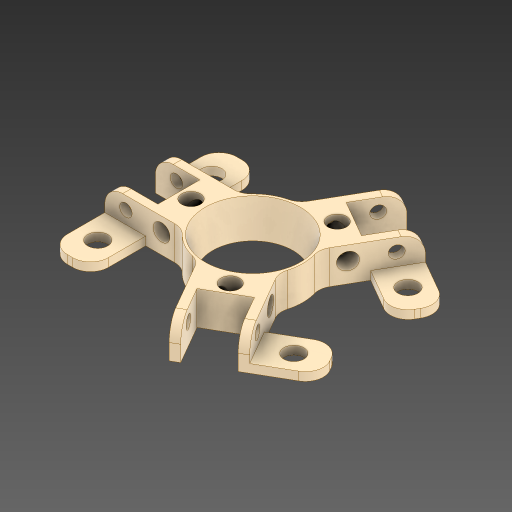
# Autodesk Inventor part: Base v6
Saved by Autodesk Inventor 2024 (Build 280153000, 153)
## iProperties
Created: 2024-01-11
Part Number: Base v6
Material: PC/ABS Plastic
Document SubType Name: Modeling
Designer: czb556
Density: 1.1 g/cm^3
Appearance: Smooth - Off-White
Author: czb556
## iProperties of the stored document Base v6_3DPrint.ipt
Created: 2024-01-12
Part Number: Base v6_3DPrint
Material: Generic
Document SubType Name: Modeling
Designer: baloc
Density: 1 g/cm^3
Appearance: Default
Author: baloc
Autodesk Inventor part; units mm, degrees
ref_plane "YZ Plane" through (0, 0, 0) normal (1, 0, 0) x (0, 1, 0)
ref_plane "XZ Plane" through (0, 0, 0) normal (0, 1, 0) x (-1, 0, 0)
ref_plane "XY Plane" through (0, 0, 0) normal (0, 0, 1) x (1, 0, 0)
sketch "Nut/Rod Template" plane through (0, 0, 0) normal (0, 1, 0) x (-1, 0, 0)
  line L0 (0, 0) -> (22, 0) construction
  line L1 (-34.925, -20.32) -> (34.925, -20.32)
  line L2 (34.925, -20.32) -> (34.925, 20.32)
  line L3 (34.925, 20.32) -> (-34.925, 20.32)
  line L4 (-34.925, 20.32) -> (-34.925, -20.32)
  line L5 (-34.925, -20.32) -> (34.925, 20.32) construction
  line L6 (34.925, -20.32) -> (-34.925, 20.32) construction
  line L7 (34.925, -26.909) -> (29.2188, -23.6145)
  line L8 (29.2188, -23.6145) -> (29.2188, -17.0255)
  line L9 (29.2188, -17.0255) -> (34.925, -13.731)
  line L10 (34.925, -13.731) -> (40.6312, -17.0255)
  line L11 (40.6312, -17.0255) -> (40.6312, -23.6145)
  line L12 (40.6312, -23.6145) -> (34.925, -26.909)
  line L13 (29.2187, 23.6145) -> (34.925, 26.909)
  line L14 (34.925, 26.909) -> (40.6312, 23.6145)
  line L15 (40.6312, 23.6145) -> (40.6312, 17.0255)
  line L16 (40.6312, 17.0255) -> (34.925, 13.731)
  line L17 (34.925, 13.731) -> (29.2188, 17.0255)
  line L18 (29.2188, 17.0255) -> (29.2187, 23.6145)
  line L19 (-40.6312, -17.0255) -> (-34.925, -13.731)
  line L20 (-34.925, -13.731) -> (-29.2188, -17.0255)
  line L21 (-29.2188, -17.0255) -> (-29.2188, -23.6145)
  line L22 (-29.2188, -23.6145) -> (-34.925, -26.909)
  line L23 (-34.925, -26.909) -> (-40.6312, -23.6145)
  line L24 (-40.6312, -23.6145) -> (-40.6312, -17.0255)
  line L25 (-40.6313, 23.6145) -> (-34.925, 26.909)
  line L26 (-34.925, 26.909) -> (-29.2188, 23.6145)
  line L27 (-29.2188, 23.6145) -> (-29.2188, 17.0255)
  line L28 (-29.2188, 17.0255) -> (-34.925, 13.731)
  line L29 (-34.925, 13.731) -> (-40.6313, 17.0255)
  line L30 (-40.6313, 17.0255) -> (-40.6313, 23.6145)
  dimension "d6" = 22
  dimension "d24" = 40.64
  dimension "d25" = 69.85
  dimension "d60" = 11.4125
  dimension "d63" = 40.64
  dimension "d66" = 69.85
  constraints: 62 end point, 3 horizontal, 2 coincident, 2 midpoint, 2 parallel, 1 perpendicular, 1 point on line, 1 vertical, 49 other
  measures "d6" distance of L0.start L0.end
  measures "d24" distance of L1.end L2.end
  measures "d25" distance of L2.end L3.end
  measures "d60" distance between parallel lines of L7 L10
  measures "d63" distance of L8.end L13.start
  measures "d66" distance of L8.end L19.start
sketch "Sketch2" plane through (0, 0, 0) normal (0, 1, 0) x (-1, 0, 0)
  line L0 (0, 0) -> (22, 0) construction
  circle A0 centre (22, 0) radius 3.325
  line L1 (26.325, 7.5) -> (42.2, 7.5)
  line L2 (42.2, -7.5) -> (26.325, -7.5)
  line L3 (42.2, 10.5) -> (14.3485, 10.5)
  line L4 (42.2, 10.5) -> (42.2, 7.5)
  line L5 (42.2, -7.5) -> (42.2, -10.5)
  line L6 (42.2, -10.5) -> (14.3485, -10.5)
  circle A1 centre (0, 0) radius 14.2875
  line L7 (26.325, 7.5) -> (26.325, -7.5)
  circle A2 centre (0, 0) radius 17.78
  line L8 (-30.1933, 31.2963) -> (-16.2675, 7.1761)
  line L9 (-19.6577, 19.0481) -> (-27.5952, 32.7963)
  line L10 (-30.1933, 31.2963) -> (-27.5952, 32.7963)
  circle A3 centre (-11, 19.0526) radius 3.325
  line L11 (-19.6577, 19.0481) -> (-6.6673, 26.5481)
  line L12 (-14.6048, 40.2963) -> (-6.6673, 26.5481)
  line L13 (-14.6048, 40.2963) -> (-12.0067, 41.7963)
  line L14 (-12.0067, 41.7963) -> (1.919, 17.6761)
  line L15 (-12.0067, -41.7963) -> (1.919, -17.6761)
  line L16 (-6.6673, -26.5481) -> (-14.6048, -40.2963)
  line L17 (-12.0067, -41.7963) -> (-14.6048, -40.2963)
  circle A4 centre (-11, -19.0526) radius 3.325
  line L18 (-6.6673, -26.5481) -> (-19.6577, -19.0481)
  line L19 (-27.5952, -32.7963) -> (-19.6577, -19.0481)
  line L20 (-27.5952, -32.7963) -> (-30.1933, -31.2963)
  line L21 (-30.1933, -31.2963) -> (-16.2675, -7.1761)
  point P0 (14.3485, 10.5)
  point P1 (1.919, 17.6761)
  dimension "d19" = 35.56
  dimension "d10" = 6.65
  dimension "d11" = 15
  dimension "d13" = 4.325
  dimension "d14" = 3
  dimension "d17" = 28.575
  dimension "d18" = 15.875
  dimension "d22" = 360
  constraints: 42 end point, 4 centre point, 3 coincident, 3 equal length, 3 vertical, 2 horizontal, 1 collinear, 1 perpendicular, 56 other
  measures "d10" diameter of A0
  measures "d11" distance of L1.end L2.start
  measures "d13" horizontal distance of L0.end L1.start
  measures "d14" distance between parallel lines of L1 L3
  measures "d17" diameter of A1
  measures "d18" distance of L1.start L1.end
extrude "Spring Holder" add sketch "Sketch2" along normal blind 12
sketch "Sketch5" plane through (30.1933, 0, -31.2963) normal (0.8660254, 0, 0.5) x (0.5, 0, -0.8660254)
  line L0 (0, 0) -> (0, 12) projected
  line L1 (-27.8515, 12) -> (0, 12) projected
  point P0 (-42.2, 0)
  point P1 (-7.5, 7.5)
  dimension "d39" = 7.5
  dimension "d40" = 4.5
  measures "d39" distance from line of L0 point (-7.5, 7.5)
  measures "d40" distance from line of L1 point (-7.5, 7.5)
hole "Spring Pin Hole" at (26.4433, 7.5, -24.8011) direction (-0.8660254, 0, -0.5) diameter 4.4 end through all
pattern_circular "Pin Pattern" count 3 over 360 about axis through (0, -10, 0) along (0, 1, 0) of "Spring Pin Hole"
sketch "Sketch12" plane through (0, 0, 0) normal (0, 1, 0) x (-1, 0, 0)
  line L0 (40.6312, 23.6145) -> (40.6312, 17.0255) projected
  line L1 (34.925, 26.909) -> (40.6312, 23.6145) projected
  line L2 (29.2187, 23.6145) -> (34.925, 26.909) projected
  line L3 (29.2188, 17.0255) -> (29.2187, 23.6145) projected
  line L4 (34.925, 13.731) -> (29.2188, 17.0255) projected
  line L5 (40.6312, 17.0255) -> (34.925, 13.731) projected
  line L6 (-29.2188, 23.6145) -> (-29.2188, 17.0255) projected
  line L7 (-34.925, 26.909) -> (-29.2188, 23.6145) projected
  line L8 (-40.6313, 23.6145) -> (-34.925, 26.909) projected
  line L9 (-40.6313, 17.0255) -> (-40.6313, 23.6145) projected
  line L10 (-34.925, 13.731) -> (-40.6313, 17.0255) projected
  line L11 (-29.2188, 17.0255) -> (-34.925, 13.731) projected
  line L12 (42.2, 10.5) -> (14.3485, 10.5) projected
  line L13 (42.2, 10.5) -> (42.2, 30.14)
  line L14 (42.2, 30.14) -> (27.65, 30.14)
  line L15 (27.65, 30.14) -> (27.65, 10.5)
  line L16 (62.9087, 0) -> (-47.4368, 0)
  line L17 (42.2, -10.5) -> (42.2, -30.14)
  line L18 (42.2, -30.14) -> (27.65, -30.14)
  line L19 (27.65, -30.14) -> (27.65, -10.5)
  line L20 (14.3485, -10.5) -> (42.2, -10.5) projected
  line L21 (-16.2675, -7.1761) -> (-30.1933, -31.2963) projected
  arc A0 (-16.2675, 7.1761) -> (-16.2675, -7.1761) centre (0, 0) ccw projected
  line L22 (-30.1933, 31.2963) -> (-16.2675, 7.1761) projected
  line L23 (-30.1933, -31.2963) -> (-27.5952, -32.7963) projected
  line L24 (-27.5952, 32.7963) -> (-30.1933, 31.2963) projected
  line L25 (-30.1933, 31.2963) -> (-46.7966, 21.7103)
  line L26 (-23.0534, 18.9297) -> (-39.6567, 9.3437)
  line L27 (-46.7966, 21.7103) -> (-39.6567, 9.3437)
  line L28 (-30.1933, -31.2963) -> (-46.7966, -21.7103)
  line L29 (-23.0534, -18.9297) -> (-39.6567, -9.3437)
  line L30 (-46.7966, -21.7103) -> (-39.6567, -9.3437)
  dimension "d93" = 1.5688
  dimension "d94" = 1.5688
  dimension "d95" = 3.231
  dimension "d96" = 3.231
  dimension "d97" = 1.4336
  dimension "d104" = 1.4336
  dimension "d107" = 2.9969
  dimension "d108" = 2.9969
  constraints: 28 end point, 7 symmetric about line, 2 parallel, 2 perpendicular, 2 point on line, 1 horizontal, 1 vertical
  measures "d93" distance between parallel lines of L13 L0
  measures "d94" distance between parallel lines of L15 L3
  measures "d95" distance from line of L12 L4.start
  measures "d96" distance from line of L14 L1.start
  measures "d97" distance between parallel lines of L25 L8
  measures "d104" distance between parallel lines of L26 L11
  measures "d107" distance from line of L22 L6.start
  measures "d108" distance from line of L27 L9.start
extrude "Plate" add sketch "Sketch12" along normal blind 3 contours L0 L5 L4 L3 L2 L1 | L6 L11 L10 L9 L8 L7 | L12 L15 L14 L13 | L17 L18 L19 L20 | L21 L28 L30 L29 | L22 L26 L27 L25
hole "MNTG Holes" at (-34.925, 0, -20.32) at (-34.925, 0, 20.32) at (34.925, 0, 20.32) at (34.925, 0, -20.32) direction (0, 1, 0) diameter 7.1374 end through all clearance for "Hex Head Bolt" size "1/4" standard "Ansi Unified Screw Threads"
fillet ".25\" Filet" radius 6.35 20 edges at (46.7966, 1.5, 21.7103) (39.6567, 1.5, 9.3437) (39.6567, 1.5, -9.3437) (46.7966, 1.5, -21.7103) (-27.65, 1.5, -30.14) (-42.2, 1.5, -30.14) (-42.2, 1.5, 30.14) (-27.65, 1.5, 30.14) (-42.2, 12, 9) (-42.2, 12, -9) (13.3058, 12, 41.0463) (28.8942, 12, 32.0463) (28.8942, 12, -32.0463) (13.3058, 12, -41.0463) (16.2675, 6, 7.1761) (16.2675, 6, -7.1761) (-1.919, 6, -17.6761) (-14.3485, 6, -10.5) (-14.3485, 6, 10.5) (-1.919, 6, 17.6761)
sketch "Sketch14" plane through (-42.2, 3, 10.5) normal (0, 0, 1) x (1, 0, 0)
  line L0 (16.875, 9) -> (23.525, 9) projected
  line L1 (16.875, -3) -> (23.525, -3) projected
  point P0 (42.2, -3)
  point P1 (20.2, 4)
  point P2 (20.2, 9)
  dimension "d118" = 5
  constraints: 1 midpoint, 1 vertical alignment
  measures "d118" distance of point (20.2, 4) point (20.2, 9)
hole "Set Screw Holes" at (-22, 7, 10.5) direction (0, 0, -1) diameter 6 end through all
draft "FaceDraft1" angle 12.5 pull direction (0, 1, 0) faces at (-14.1025, 8, -2.2919) fixed edges at (14.2875, 0, 0)
pattern_circular "Circular Pattern2" count 3 over 360 about axis through (0, 0, 0) along (0, 1, 0) of "Set Screw Holes"
body "Solid1"
